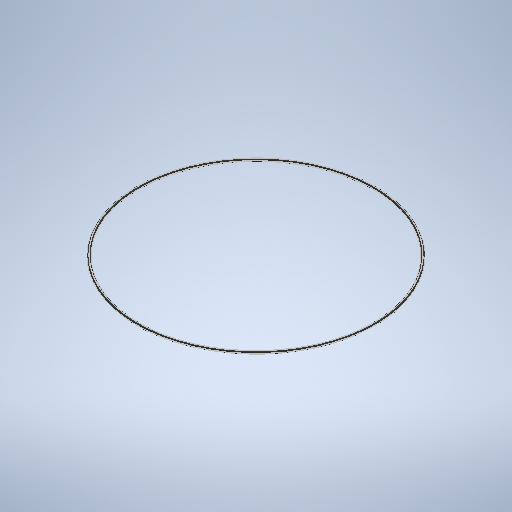
# Autodesk Inventor part: RubberSeal
Saved by Autodesk Inventor 2026.2 (Build 302298000, 298)
## iProperties
Created: 2026-03-01
Part Number: RubberSeal
Material: Rubber
Document SubType Name: Modeling
Designer: mumin
Density: 0.93 g/cm^3
Appearance: Rubber - Black
Author: mumin
Autodesk Inventor part; units mm, degrees
ref_plane "YZ Plane" through (0, 0, 0) normal (1, 0, 0) x (0, 1, 0)
ref_plane "XZ Plane" through (0, 0, 0) normal (0, 1, 0) x (-1, 0, 0)
ref_plane "XY Plane" through (0, 0, 0) normal (0, 0, 1) x (1, 0, 0)
sketch "Sketch1" plane through (0, 0, 0) normal (0, 0, 1) x (1, 0, 0)
  line L0 (0, -2.3369) -> (0, 2.3369) projected
  line L1 (115.3, -1.4) -> (115.5, -1.4)
  line L2 (116.8, -0.1) -> (116.8, 0.1)
  line L3 (115.5, 1.4) -> (115.3, 1.4)
  line L4 (114, 0.1) -> (114, -0.1)
  line L5 (114, -1.4) -> (116.8, 1.4) construction
  line L6 (116.8, -1.4) -> (114, 1.4) construction
  arc A0 (116.8, 0.1) -> (115.5, 1.4) centre (115.5, 0.1) ccw
  arc A1 (115.3, 1.4) -> (114, 0.1) centre (115.3, 0.1) ccw
  arc A2 (114, -0.1) -> (115.3, -1.4) centre (115.3, -0.1) ccw
  arc A3 (115.5, -1.4) -> (116.8, -0.1) centre (115.5, -0.1) ccw
  point P0 (0, 0)
  dimension "d4" = 114
  dimension "d5" = 1.3
  constraints: 12 end point, 8 point on circle, 8 point on line, 8 tangent, 4 centre point, 3 equal radius, 2 parallel, 1 horizontal, 1 perpendicular
  measures "d4" distance between parallel lines of L0 L4
  measures "d5" radius of A0
revolve "Rubber Seal" add sketch "Sketch1" angle 360 about axis through (0, -10, 0) along (0, 1, 0)
body "Solid1"
